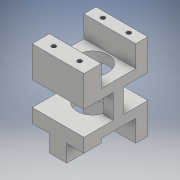
# Autodesk Inventor part: RotationShell
Saved by Autodesk Inventor 2018 (Build 220112000, 112)
## iProperties
Created: 2019-06-06
Part Number: RotationShell
Material: Generic
Document SubType Name: Modeling
Designer: aal_9
Density: 1 g/cm^3
Appearance: Default
Author: aal_9
Autodesk Inventor part; units mm, degrees
ref_plane "YZ Plane" through (0, 0, 0) normal (1, 0, 0) x (0, 1, 0)
ref_plane "XZ Plane" through (0, 0, 0) normal (0, 1, 0) x (-1, 0, 0)
ref_plane "XY Plane" through (0, 0, 0) normal (0, 0, 1) x (1, 0, 0)
sketch "Sketch1" plane through (0, 0, 0) normal (0, 0, 1) x (1, 0, 0)
  line L0 (-15, 17) -> (15, 17)
  line L1 (15, 17) -> (15, -20)
  line L2 (15, -20) -> (-15, -20)
  line L3 (-15, -20) -> (-15, 17)
  point P0 (0, 0)
  dimension "d0" = 37
  dimension "d1" = 30
  dimension "d2" = 15
  dimension "d3" = 20
  constraints: 8 end point, 2 parallel, 1 horizontal, 1 perpendicular
  measures "d0" distance of L2.end L0.start
  measures "d1" distance of L1.end L2.end
  measures "d2" distance from line of L1 point (0, 0)
  measures "d3" distance from line of point (0, 0) L2
extrude "Extrusion1" add sketch "Sketch1" along normal blind 50
sketch "Sketch2" plane through (0, 0, 50) normal (0, 0, 1) x (1, 0, 0)
  circle A0 centre (0, 0) radius 9
  dimension "d6" = 18
  constraints: 2 coincident, 1 centre point
  measures "d6" diameter of A0
extrude "Extrusion2" cut sketch "Sketch2" against normal through all
sketch "Sketch3" plane through (15, -20, 0) normal (1, 0, 0) x (0, 0, -1)
  line L0 (-50, 30) -> (-37.5, 30)
  line L1 (-37.5, 30) -> (-37.5, 10)
  line L2 (-37.5, 10) -> (-50, 10)
  line L3 (-50, 10) -> (-50, 30)
  line L4 (0, 0) -> (0, 37) projected
  line L5 (0, 30) -> (-12.5, 30)
  line L6 (-12.5, 30) -> (-12.5, 10)
  line L7 (-12.5, 10) -> (0, 10)
  line L8 (0, 10) -> (0, 30)
  line L9 (0, 0) -> (-50, 0) projected
  line L10 (0, 37) -> (-50, 37) projected
  line L11 (-50, 0) -> (-50, 37) projected
  point P0 (0, 20)
  dimension "d9" = 10
  dimension "d10" = 7
  dimension "d11" = 10
  dimension "d12" = 0
  dimension "d13" = 12.5
  dimension "d14" = 12.5
  constraints: 16 end point, 4 parallel, 2 horizontal, 2 perpendicular, 2 point on line
  measures "d9" distance between parallel lines of L9 L2
  measures "d10" distance between parallel lines of L10 L0
  measures "d11" distance between parallel lines of L9 L7
  measures "d12" distance between parallel lines of L11 L3
  measures "d13" distance between parallel lines of L3 L1
  measures "d14" distance between parallel lines of L4 L6
extrude "Extrusion3" cut sketch "Sketch3" against normal through all contours L0 L1 L2 L3 | L4 L7 L6 L5
sketch "Sketch4" plane through (15, -20, 50) normal (1, 0, 0) x (0, 0, -1)
  line L0 (18, 37) -> (32, 37)
  line L1 (32, 37) -> (32, 23)
  line L2 (32, 23) -> (18, 23)
  line L3 (18, 23) -> (18, 37)
  line L4 (18, 0) -> (32, 0)
  line L5 (32, 0) -> (32, 17)
  line L6 (32, 17) -> (18, 17)
  line L7 (18, 17) -> (18, 0)
  line L8 (50, 37) -> (0, 37) projected
  line L9 (50, 0) -> (0, 0) projected
  line L10 (0, 30) -> (0, 37) projected
  point P0 (50, 20)
  dimension "d17" = 14
  dimension "d18" = 0
  dimension "d19" = 0
  dimension "d20" = 18
  dimension "d21" = 17
  dimension "d22" = 14
  constraints: 16 end point, 4 parallel, 2 horizontal, 2 perpendicular, 2 point on line
  measures "d17" distance of L0.start L0.end
  measures "d18" distance between parallel lines of L8 L0
  measures "d19" distance between parallel lines of L9 L4
  measures "d20" distance between parallel lines of L10 L3
  measures "d21" distance of L4.end L5.end
  measures "d22" distance of L0.end L1.end
extrude "Extrusion4" cut sketch "Sketch4" against normal through all
sketch "Sketch5" plane through (0, 0, 0) normal (0, 0, -1) x (-1, 0, 0)
  line L0 (-15, -20) -> (15, -20) projected
  line L1 (-15, -20) -> (-5, -20)
  line L2 (-5, -20) -> (-5, -10)
  line L3 (-5, -10) -> (-15, -10)
  line L4 (-15, -10) -> (-15, -20)
  line L5 (15, -20) -> (5, -20)
  line L6 (5, -20) -> (5, -10)
  line L7 (5, -10) -> (15, -10)
  line L8 (15, -10) -> (15, -20)
  line L9 (15, -10) -> (-15, -10) projected
  point P0 (0, 0)
  dimension "d27" = 10
  dimension "d28" = 10
  dimension "d31" = 0
  dimension "d32" = 0
  constraints: 16 end point, 4 parallel, 2 horizontal, 2 perpendicular
  measures "d27" distance between parallel lines of L8 L6
  measures "d28" distance between parallel lines of L4 L2
  measures "d31" distance between parallel lines of L3 L9
  measures "d32" distance between parallel lines of L7 L9
extrude "Extrusion5" cut sketch "Sketch5" against normal blind 10 contours L4 L3 L2 L0 | L6 L7 L8 L0
sketch "Sketch6" plane through (0, 0, 50) normal (0, 0, 1) x (1, 0, 0)
  line L0 (15, 17) -> (-15, 17) projected
  line L1 (-15, 17) -> (-15, 10) projected
  line L2 (-15, -10) -> (-15, -20) projected
  line L3 (-15, -20) -> (15, -20) projected
  point P0 (0, 0)
  point P1 (-7.5, 13.5)
  point P2 (7.5, 13.5)
  point P3 (-7.5, -15)
  point P4 (7.5, -15)
  dimension "d33" = 3.5
  dimension "d34" = 3.5
  dimension "d35" = 15
  dimension "d36" = 7.5
  dimension "d37" = 7.5
  dimension "d38" = 15
  dimension "d39" = 5
  dimension "d40" = 5
  measures "d33" distance from line of L0 point (-7.5, 13.5)
  measures "d34" distance from line of L0 point (7.5, 13.5)
  measures "d35" distance of point (-7.5, 13.5) point (7.5, 13.5)
  measures "d36" distance from line of L1 point (-7.5, 13.5)
  measures "d37" distance from line of L2 point (-7.5, -15)
  measures "d38" distance of point (7.5, -15) point (-7.5, -15)
  measures "d39" distance from line of L3 point (7.5, -15)
  measures "d40" distance from line of L3 point (-7.5, -15)
hole "Hole1" at (-7.5, 13.5, 50) at (7.5, 13.5, 50) at (-7.5, -15, 50) at (7.5, -15, 50) direction (0, 0, -1) diameter 2.459 depth 8 tip angle 118 thread size "M3x0.5" class "6H" standard "ANSI Metric M Profile"
sketch "Sketch7" plane through (0, 0, 0) normal (0, 0, -1) x (-1, 0, 0)
  circle A0 centre (-7.5, 13.5) radius 1.2295 projected
  circle A1 centre (7.5, 13.5) radius 1.2295 projected
  point P0 (0, 0)
  point P1 (0, -15)
  dimension "d49" = 15
  dimension "d50" = 0
  constraints: 2 coincident
  measures "d49" distance of point (0, -15) point (0, 0)
  measures "d50" horizontal distance of point (0, 0) point (0, -15)
hole "Hole2" at (7.5, 13.5, 0) at (-7.5, 13.5, 0) at (0, -15, 0) direction (0, 0, 1) diameter 2.459 depth 8 tip angle 118 thread size "M3x0.5" class "6H" standard "ANSI Metric M Profile"
sketch "Sketch8" plane through (-15, 3, 18) normal (0, 1, 0) x (1, 0, 0)
  line L0 (30, -14) -> (23.4853, -14) projected
  line L1 (5.5147, 0) -> (24.4853, 0)
  line L2 (24.4853, 0) -> (24.4853, -14)
  line L3 (24.4853, -14) -> (5.5147, -14)
  line L4 (5.5147, -14) -> (5.5147, 0)
  line L5 (0, 0) -> (30, 0) projected
  line L6 (23.4853, -14) -> (23.4853, 0) projected
  line L7 (6.5147, 0) -> (6.5147, -14) projected
  point P0 (15, 18)
  dimension "d58" = 0
  dimension "d59" = 1
  dimension "d60" = 1
  constraints: 8 end point, 2 parallel, 1 horizontal, 1 perpendicular, 1 point on line
  measures "d58" distance between parallel lines of L5 L1
  measures "d59" distance between parallel lines of L6 L2
  measures "d60" distance between parallel lines of L7 L4
extrude "Extrusion6" cut sketch "Sketch8" against normal through all contours L0 L6 L1 L2 | L3 L4 L1 L7
body "Solid1"
